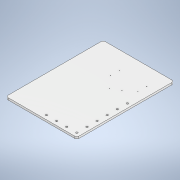
# Autodesk Inventor part: bottom_plate
Saved by Autodesk Inventor 2021.3 (Build 253353010, 353A)
## iProperties
Created: 2022-03-04
Part Number: bottom_plate
Material: Acetal Resin, White
Document SubType Name: Modeling
Designer: au504769
Density: 1.425 g/cm^3
Appearance: Smooth - White
Author: au504769
Autodesk Inventor part; units mm, degrees
ref_plane "YZ Plane" through (0, 0, 0) normal (1, 0, 0) x (0, 1, 0)
ref_plane "XZ Plane" through (0, 0, 0) normal (0, 1, 0) x (-1, 0, 0)
ref_plane "XY Plane" through (0, 0, 0) normal (0, 0, 1) x (1, 0, 0)
sketch "Sketch1" plane through (0, 0, 0) normal (0, 1, 0) x (-1, 0, 0)
  line L0 (0, 0) -> (350, 0)
  line L1 (350, 0) -> (350, -480)
  line L2 (350, -480) -> (0, -480)
  line L3 (0, -480) -> (0, 0)
  dimension "d0" = 480
  dimension "d1" = 350
  constraints: 8 end point, 2 parallel, 1 horizontal, 1 perpendicular
  measures "d0" distance between parallel lines of L2 L0
  measures "d1" distance between parallel lines of L1 L3
extrude "Extrusion1" add sketch "Sketch1" along normal blind 10
fillet "Fillet1" radius 10 4 edges at (-350, 5, 0) (0, 5, 0) (0, 5, -480) (-350, 5, -480)
sketch "Sketch5" plane through (0, 0, 0) normal (0, 1, 0) x (-1, 0, 0)
  line L0 (340, 0) -> (10, 0) projected
  line L1 (0, -10) -> (0, -470) projected
  line L2 (20, -70) -> (20, -170) construction
  line L3 (20, -120) -> (20, -220) construction
  line L4 (20, -170) -> (20, -270) construction
  line L5 (20, -20) -> (120, -20) construction
  line L6 (20, -20) -> (20, -120) construction
  line L7 (170, -20) -> (70, -20) construction
  point P0 (0, 0)
  dimension "d32" = 100
  dimension "d33" = 70
  dimension "d34" = 20
  dimension "d43" = 50
  constraints: 12 end point, 5 equal length, 4 vertical alignment, 3 vertical, 1 collinear, 1 horizontal, 1 horizontal alignment, 1 midpoint, 1 point on line
  measures "d32" distance of L2.start L2.end
  measures "d33" distance from line of L2.start L0
  measures "d34" distance from line of L2.start L1
  measures "d43" distance of L2.start L3.start
hole "Hole4" at (-170, 0, -20) at (-120, 0, -20) at (-70, 0, -20) at (-20, 0, -20) at (-20, 0, -70) at (-20, 0, -120) at (-20, 0, -170) at (-20, 0, -220) at (-20, 0, -270) direction (0, 1, 0) diameter 9 end through all countersink diameter 17.3 countersink angle 90 clearance for "Countersunk Flat Head Screw ISO 2009/7046" size "M8" standard "ISO"
sketch "Sketch2" plane through (0, 0, 0) normal (0, 1, 0) x (-1, 0, 0)
  line L0 (0, -10) -> (0, -470) projected
  line L1 (10, -480) -> (340, -480) projected
  line L2 (88.75, -311.5) -> (108.75, -311.5) construction
  line L3 (108.75, -311.5) -> (128.75, -311.5) construction
  line L4 (108.75, -311.5) -> (112.75, -346.5) construction
  line L5 (45, -346.5) -> (112.75, -346.5) construction
  line L6 (180.5, -346.5) -> (112.75, -346.5) construction
  point P0 (0, 0)
  point P1 (45, -390)
  point P2 (180.5, -390)
  point P3 (128.75, -290.5)
  dimension "d20" = 43.5
  dimension "d21" = 135.5
  dimension "d22" = 45
  dimension "d23" = 90
  dimension "d26" = 40
  dimension "d28" = 21
  dimension "d30" = 35
  dimension "d31" = 4
  constraints: 10 end point, 3 collinear, 3 horizontal alignment, 3 vertical alignment, 2 horizontal, 1 point on line
  measures "d20" distance of point (45, -390) L5.start
  measures "d21" distance of point (180.5, -390) point (45, -390)
  measures "d22" distance from line of L0 point (45, -390)
  measures "d23" distance from line of L1 point (45, -390)
  measures "d26" horizontal distance of point (128.75, -290.5) L2.start
  measures "d28" vertical distance of L2.start point (128.75, -290.5)
  measures "d30" vertical distance of L4.end L2.end
  measures "d31" horizontal distance of L4.end L2.end
hole "Hole5" at (-128.75, 0, -290.5) at (-88.75, 0, -311.5) at (-180.5, 0, -346.5) at (-180.5, 0, -390) at (-45, 0, -346.5) at (-45, 0, -390) direction (0, 1, 0) diameter 2.459 end through all thread size "M3x0.5" class "6H" standard "ISO Metric profile"
sketch "Sketch3" plane through (0, 0, 0) normal (0, 1, 0) x (-1, 0, 0)
  line L0 (350, -470) -> (350, -10) construction
  line L1 (350, -20) -> (330, -20) construction
  line L2 (330, -20) -> (330, 0) construction
  line L3 (0, -10) -> (0, -470) construction
  line L4 (0, -20) -> (20, -20) construction
  line L5 (20, -20) -> (20, 0) construction
  line L6 (340, 0) -> (10, 0) construction
  line L7 (0, -460) -> (20, -460) construction
  line L8 (20, -460) -> (20, -480) construction
  line L9 (10, -480) -> (340, -480) construction
  line L10 (330, -480) -> (330, -460) construction
  line L11 (330, -460) -> (350, -460) construction
  point P0 (0, 0)
  dimension "d12" = 20
  constraints: 16 end point, 8 point on line, 7 equal length, 4 perpendicular, 3 horizontal, 1 vertical
  measures "d12" distance of L10.end L11.end
body "Solid1"
